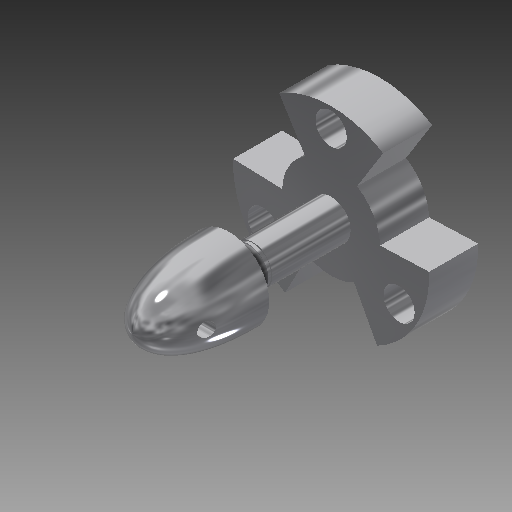
# Autodesk Inventor part: HK 2830 1100 prop adapter
Saved by Autodesk Inventor 2019 (Build 230136000, 136)
## iProperties
Created: 2014-01-15
Part Number: HK 2830 1100 prop adapter
Document SubType Name: Modeling
Designer: Phil
Density: 1 g/cm^3
Material: Generic
Appearance: Aluminum - Polished
Author: Phil
Autodesk Inventor part; units mm, degrees
ref_plane "YZ Plane" through (0, 0, 0) normal (1, 0, 0) x (0, 1, 0)
ref_plane "XZ Plane" through (0, 0, 0) normal (0, 1, 0) x (-1, 0, 0)
ref_plane "XY Plane" through (0, 0, 0) normal (0, 0, 1) x (1, 0, 0)
sketch "Sketch1" plane through (0, 0, 0) normal (0, 0, 1) x (1, 0, 0)
  circle A0 centre (0, 0) radius 4
  circle A1 centre (0, 0) radius 10
  circle A2 centre (-6.9282, -4) radius 1.0065 projected
  circle A3 centre (6.9282, -4) radius 1.0065 projected
  circle A4 centre (0, 8) radius 1.0065 projected
  dimension "d0" = 8
  dimension "d1" = 20
  constraints: 2 centre point, 2 coincident
  measures "d0" diameter of A0
  measures "d1" diameter of A1
extrude "Extrusion1" add sketch "Sketch1" along normal blind 5
sketch "Sketch2" plane through (0, 0, 5) normal (0, 0, 1) x (1, 0, 0)
  circle A0 centre (0, 0) radius 4 projected
  circle A1 centre (0, 0) radius 10 projected
  line L0 (3.9976, 0.1396) -> (13.5917, 0.4746) projected
  line L1 (7.2069, 11.5335) -> (2.1197, 3.3922) projected
  line L2 (3.9976, 0.1396) -> (6.6264, 0.2314)
  line L3 (9.9939, 0.349) -> (5.2992, 8.4805)
  line L4 (9.9939, 0.349) -> (3.9976, 0.1396)
  line L5 (2.1197, 3.3922) -> (5.2992, 8.4805)
  arc A2 (3.9976, 0.1396) -> (2.1197, 3.3922) centre (0, 0) ccw
  arc A3 (9.9939, 0.349) -> (5.2992, 8.4805) centre (0, 0) ccw
  constraints: 8 end point, 6 point on circle, 3 point on line, 2 centre point, 2 collinear, 2 concentric
extrude "Extrusion2" cut sketch "Sketch2" against normal blind 5 contours A0 L1 L3 L0 | A1 L3
pattern_circular "Circular Pattern1" count 3 over 360 about axis through (0, 0, 0) along (0, 0, 1) of "Extrusion2"
sketch "Sketch3" plane through (0, 0, 5) normal (0, 0, 1) x (1, 0, 0)
  arc A0 (-9.9939, 0.349) -> (-4.6947, -8.8295) centre (0, 0) ccw projected
  circle A1 centre (0, 0) radius 5
  dimension "d9" = 10
  constraints: 1 centre point, 1 coincident
  measures "d9" diameter of A1
extrude "Extrusion3" add sketch "Sketch3" against normal blind 5
sketch "Sketch4" plane through (0, 0, 5) normal (0, 0, 1) x (1, 0, 0)
  circle A0 centre (6.9282, -4) radius 1.0065 projected
  circle A1 centre (0, 8) radius 1.0065 projected
  circle A2 centre (-6.9282, -4) radius 1.0065 projected
  circle A3 centre (-6.9282, -4) radius 1.6
  circle A4 centre (6.9282, -4) radius 1.6
  circle A5 centre (0, 8) radius 1.6
  dimension "d12" = 3.2
  dimension "d13" = 3.2
  dimension "d14" = 3.2
  constraints: 3 centre point, 3 coincident
  measures "d12" diameter of A4
  measures "d13" diameter of A3
  measures "d14" diameter of A5
extrude "Extrusion4" cut sketch "Sketch4" against normal blind 3
sketch "Sketch5" plane through (0, 0, 5) normal (0, 0, 1) x (1, 0, 0)
  arc A0 (-9.9939, 0.349) -> (-4.6947, -8.8295) centre (0, 0) ccw projected
  circle A1 centre (0, 0) radius 2
  dimension "d17" = 4
  constraints: 1 centre point, 1 coincident
  measures "d17" diameter of A1
extrude "Extrusion5" add sketch "Sketch5" along normal blind 8
sketch "Sketch6" plane through (0, 0, 13) normal (0, 0, 1) x (1, 0, 0)
  circle A0 centre (0, 0) radius 2 projected
  circle A1 centre (0, 0) radius 1.9
  dimension "d20" = 3.8
  constraints: 1 centre point, 1 coincident
  measures "d20" diameter of A1
extrude "Extrusion6" add sketch "Sketch6" along normal blind 0.4 contours A1
sketch "Sketch7" plane through (0, 0, 13.4) normal (0, 0, 1) x (1, 0, 0)
  circle A0 centre (0, 0) radius 1.9 projected
  circle A1 centre (0, 0) radius 2
  dimension "d23" = 4
  constraints: 1 centre point, 1 coincident
  measures "d23" diameter of A1
extrude "Extrusion7" add sketch "Sketch7" along normal blind 10 contours A0 | A1
thread "Thread1" size "M4x0.7" class "6g" standard "ANSI Metric M Profile" full length
chamfer "Chamfer1" distance 0.4 angle 45 1 edges at (-2, 0, 23.4)
sketch "Sketch8" plane through (0, 0, 0) normal (0, 1, 0) x (-1, 0, 0)
  line L0 (-1.6, 23.4) -> (1.6, 23.4) projected
  line L1 (0, 25.3241) -> (0, 15.4)
  line L2 (0, 15.4) -> (4.0898, 15.4)
  spline S0 degree 3 poles (0, 25.3241) (0.1432, 25.2864) (2.524, 24.659) (3.9837, 20.08) (4.062, 16.6285) (4.0898, 15.4) knots 0 0 0 0 0.044151 0.734206 1.11559 1.11559 1.11559 1.11559
  point P0 (0, 0)
  point P1 (0.4244, 25.2023)
  point P2 (3.8385, 19.2055)
  dimension "d32" = 8
  dimension "d33" = 9.9241
  constraints: 4 end point, 2 perpendicular, 4 other
  measures "d32" distance between parallel lines of L2 L0
  measures "d33" distance from line of L2 L1.start
revolve "Revolution1" add sketch "Sketch8" angle 360 about axis through (0, 0, 25.3241) along (0, 0, -1)
sketch "Sketch9" plane through (0, 0, 0) normal (1, 0, 0) x (0, 1, 0)
  line L0 (-4.0898, 15.4) -> (4.0898, 15.4) projected
  line L1 (0, 15.4) -> (0, 21.1198)
  circle A0 centre (0, 21.1198) radius 0.75
  point P0 (0, 0)
  dimension "d34" = 1.5
  constraints: 2 end point, 1 centre point, 1 coincident, 1 perpendicular
  measures "d34" diameter of A0
extrude "Extrusion8" cut sketch "Sketch9" against normal mid plane 20
equation "\"d13\" = d12"
equation "\"d14\" = d13"
body "Solid1"
